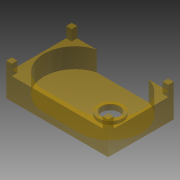
# Autodesk Inventor part: carcasatras
Saved by Autodesk Inventor 2014 SP1 (Build 180222100, 222)
## iProperties
Created: 2017-09-25
Part Number: carcasatras
Material: Generic
Document SubType Name: Modeling
Designer: Vivi
Density: 1 g/cm^3
Appearance: Oil
Author: Vivi
Autodesk Inventor part; units mm, degrees
ref_plane "YZ Plane" through (0, 0, 0) normal (1, 0, 0) x (0, 1, 0)
ref_plane "XZ Plane" through (0, 0, 0) normal (0, 1, 0) x (-1, 0, 0)
ref_plane "XY Plane" through (0, 0, 0) normal (0, 0, 1) x (1, 0, 0)
sketch "Sketch1" plane through (0, 0, 0) normal (0, 0, 1) x (1, 0, 0)
  circle A0 centre (-16.125, 0) radius 6
  arc A1 (16.125, -18.735) -> (5.2413, -15.2494) centre (10.125, -18.735) ccw
  arc A2 (16.125, 18.735) -> (5.2413, 15.2494) centre (10.125, 18.735) ccw
  circle A3 centre (10.125, 18.735) radius 7.5
  circle A4 centre (10.125, -18.735) radius 7.5
  line L0 (16.125, 27.25) -> (-16.125, 27.25)
  arc A5 (-16.125, 27.25) -> (-16.125, -27.25) centre (-16.125, 0) ccw
  line L1 (-16.125, -27.25) -> (16.125, -27.25)
  arc A6 (16.125, -27.25) -> (16.125, 27.25) centre (16.125, 0) ccw
  arc A7 (-29.2589, 27.25) -> (-16.125, -30.25) centre (-16.125, 0) ccw
  line L2 (-16.125, -30.25) -> (16.125, -30.25)
  arc A8 (16.125, -30.25) -> (29.2589, 27.25) centre (16.125, 0) ccw
  line L3 (-16.125, -30.25) -> (16.125, -30.25)
  line L4 (46.375, -30.25) -> (46.375, 27.25)
  line L5 (-46.375, 27.25) -> (-46.375, -30.25)
  line L6 (-46.375, -30.25) -> (46.375, 30.25) construction
  line L7 (46.375, -30.25) -> (-46.375, 30.25) construction
  line L8 (46.375, 27.25) -> (-46.375, 27.25)
  line L9 (-16.125, -30.25) -> (16.125, -30.25)
  line L10 (46.375, -30.25) -> (46.375, -32.25)
  line L11 (46.375, -32.25) -> (-46.375, -32.25)
  line L12 (-46.375, -32.25) -> (-46.375, -30.25)
  line L13 (-46.375, 27.25) -> (46.375, 27.25)
  line L14 (46.375, 27.25) -> (46.375, -32.25)
  line L15 (46.375, -32.25) -> (-46.375, -32.25)
  line L16 (-46.375, -32.25) -> (-46.375, 27.25)
  point P0 (0, 0)
  point P1 (0, 26.25)
  point P2 (0, -26.25)
  dimension "d1" = 12
  dimension "d3" = 12
  dimension "d4" = 12
  dimension "d6" = 15
  dimension "d7" = 15
  dimension "d9" = 3
  dimension "d12" = 2
  constraints: 34 end point, 12 point on circle, 9 centre point, 5 parallel, 4 perpendicular, 3 coincident, 3 horizontal, 3 vertical alignment, 2 midpoint, 2 point on line, 1 horizontal alignment
  measures "d1" diameter of A0
  measures "d3" diameter of A1
  measures "d4" diameter of A2
  measures "d6" diameter of A3
  measures "d7" diameter of A4
  measures "d9" radial gap between concentric circles of A8 A6
  measures "d12" distance of L10.start L10.end
extrude "Extrusion2" add sketch "Sketch1" along normal mid plane 40 contours A0 | A3 | A4 | A6 L1 A5 L0 | L8 A8 L2 A7 A5 L1 A6 | L8 L4 A8 | A7 L5 L8 | L4 L10 L11 L12 L5 A7 L2 A8
extrude "Extrusion3" cut sketch "Sketch1" along normal mid plane 36 contours A6 L1 A5 L0
extrude "Extrusion4" cut sketch "Sketch1" along normal mid plane 36 contours A0 | A3 | A4
sketch "Sketch2" plane through (0, 0, 20) normal (0, 0, 1) x (1, 0, 0)
  arc A0 (16.125, -18.735) -> (5.2413, -15.2494) centre (10.125, -18.735) ccw projected
  circle A1 centre (10.125, 18.735) radius 7.5 projected
  circle A2 centre (-16.125, 0) radius 6 projected
  circle A3 centre (10.125, 18.735) radius 7.5
  circle A4 centre (10.125, 18.735) radius 10.5
  circle A5 centre (10.125, -18.735) radius 7.5
  circle A6 centre (10.125, -18.735) radius 10.5
  circle A7 centre (-16.125, 0) radius 1.65
  circle A8 centre (-16.125, 0) radius 3.5
  point P0 (0, 0)
  point P1 (16.125, 0)
  dimension "d19" = 21
  dimension "d20" = 15
  dimension "d21" = 21
  dimension "d22" = 3.3
  dimension "d23" = 7
  constraints: 6 centre point, 6 coincident, 1 concentric
  measures "d19" diameter of A4
  measures "d20" diameter of A5
  measures "d21" diameter of A6
  measures "d22" diameter of A7
  measures "d23" diameter of A8
extrude "Extrusion5" add sketch "Sketch2" against normal blind 7 contours A4 | A6 | A8
sketch "Sketch3" plane through (0, 0, -20) normal (0, 0, -1) x (-1, 0, 0)
  circle A0 centre (-16.125, 0) radius 8.1
  circle A1 centre (-16.125, 0) radius 11.1
  point P0 (0, 0)
  dimension "d26" = 16.2
  dimension "d27" = 3
  constraints: 2 centre point, 1 coincident
  measures "d26" diameter of A0
  measures "d27" radial gap between concentric circles of A0 A1
extrude "Extrusion6" add sketch "Sketch3" against normal blind 5
extrude "Extrusion7" cut sketch "Sketch3" against normal blind 5 contours A0
extrude "Extrusion8" cut sketch "Sketch1" along normal blind 100 contours A0 | A3 | A4 | A6 L1 A5 L0 | L8 A8 L2 A7 A5 L1 A6 | L8 L4 A8 | A7 L5 L8 | L4 L10 L11 L12 L5 A7 L2 A8
sketch "Sketch4" plane through (3.9813, 27.25, 20) normal (0, -1, 0) x (1, 0, 0)
  line L0 (12.2873, -7) -> (12.2873, 0) projected
  line L1 (0, 0) -> (12.2873, 0) projected
  line L2 (0, -7) -> (0, 0) projected
  line L3 (0, -7) -> (12.2873, -7) projected
  point P0 (-3.9813, -20)
extrude "Extrusion9" cut sketch "Sketch4" against normal blind 100
sketch "Sketch5" plane through (0, 0, 0) normal (0, 0, 1) x (1, 0, 0)
  line L0 (-46.375, 27.25) -> (-41.375, 27.25)
  line L1 (-41.375, 27.25) -> (-41.375, 22.25)
  line L2 (-41.375, 22.25) -> (-46.375, 22.25)
  line L3 (-46.375, 22.25) -> (-46.375, 27.25)
  line L4 (46.375, 27.25) -> (41.375, 27.25)
  line L5 (41.375, 27.25) -> (41.375, 22.25)
  line L6 (41.375, 22.25) -> (46.375, 22.25)
  line L7 (46.375, 22.25) -> (46.375, 27.25)
  line L8 (46.375, -32.25) -> (41.375, -32.25)
  line L9 (41.375, -32.25) -> (41.375, -27.25)
  line L10 (41.375, -27.25) -> (46.375, -27.25)
  line L11 (46.375, -27.25) -> (46.375, -32.25)
  line L12 (-46.375, -32.25) -> (-41.375, -32.25)
  line L13 (-41.375, -32.25) -> (-41.375, -27.25)
  line L14 (-41.375, -27.25) -> (-46.375, -27.25)
  line L15 (-46.375, -27.25) -> (-46.375, -32.25)
  point P0 (0, 0)
  dimension "d36" = 5
  dimension "d37" = 5
  dimension "d38" = 5
  dimension "d39" = 5
  dimension "d40" = 5
  dimension "d41" = 5
  dimension "d42" = 5
  dimension "d43" = 5
  constraints: 32 end point, 8 parallel, 4 horizontal, 4 perpendicular
  measures "d36" distance of L1.end L2.end
  measures "d37" distance of L0.end L1.end
  measures "d38" distance of L6.end L5.end
  measures "d39" distance of L5.end L4.end
  measures "d40" distance of L9.end L10.end
  measures "d41" distance of L8.end L9.end
  measures "d42" distance of L14.end L13.end
  measures "d43" distance of L13.end L12.end
extrude "Extrusion10" add sketch "Sketch5" along normal blind 9.7
sketch "Sketch6" plane through (0, 0, 0) normal (0, 0, 1) x (1, 0, 0)
  arc A0 (16.125, -27.25) -> (16.125, 27.25) centre (16.125, 0) ccw projected
  line L0 (-16.125, -27.25) -> (16.125, -27.25) projected
  arc A1 (-16.125, 27.25) -> (-16.125, -27.25) centre (-16.125, 0) ccw projected
  line L1 (41.375, -32.25) -> (41.375, -27.25) projected
  line L2 (-16.125, -27.75) -> (16.125, -27.75)
  arc A2 (16.125, -27.25) -> (0, 21.9669) centre (16.125, 0) ccw
  arc A3 (0, -21.9669) -> (0.4264, -22.2736) centre (16.125, 0) ccw
  arc A4 (16.125, -27.75) -> (0, 22.5842) centre (16.125, 0) ccw
  arc A5 (-0.4264, -22.2736) -> (0, -22.5842) centre (16.125, 0) ccw
  arc A6 (0, -22.5842) -> (0.4264, -22.2736) centre (-16.125, 0) ccw
  arc A7 (0, 22.5842) -> (-16.125, -27.75) centre (-16.125, 0) ccw
  arc A8 (-0.4264, -22.2736) -> (0, -21.9669) centre (-16.125, 0) ccw
  arc A9 (0, 21.9669) -> (-16.125, -27.25) centre (-16.125, 0) ccw
  line L3 (-16.125, -28.25) -> (16.125, -28.25)
  arc A10 (16.125, -28.25) -> (0, 23.1958) centre (16.125, 0) ccw
  arc A11 (0, 23.1958) -> (-16.125, -28.25) centre (-16.125, 0) ccw
  point P0 (0, 0)
  dimension "d48" = 0.5
  constraints: 20 point on circle, 10 centre point, 6 end point, 4 coincident, 1 perpendicular, 1 tangent, 2 other
  measures "d48" radial gap between concentric circles of A11 A7
extrude "Extrusion11" cut sketch "Sketch6" against normal blind 18 contours A7 A4 L2 | A11 A10 L3
body "Solid2"
